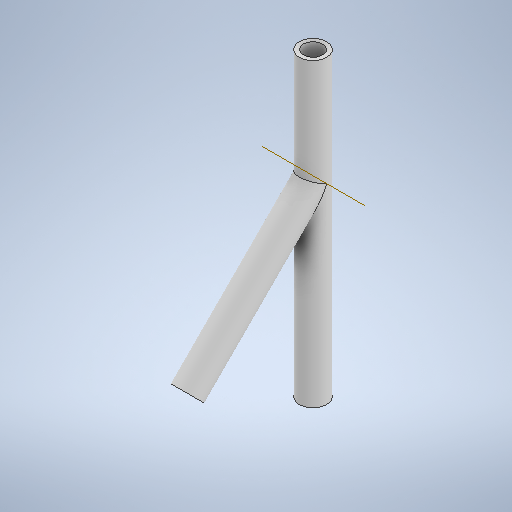
# Autodesk Inventor part: rurka
Saved by Autodesk Inventor 2025 (Build 290162000, 162)
## iProperties
Created: 2024-12-31
Part Number: rurka
Material: Ogólny
Document SubType Name: Modeling
Designer: Laptop
Density: 1 g/cm^3
Appearance: Domyślna
Author: Laptop
Autodesk Inventor part; units mm, degrees
ref_plane "YZ Plane" through (0, 0, 0) normal (1, 0, 0) x (0, 1, 0)
ref_plane "XZ Plane" through (0, 0, 0) normal (0, 1, 0) x (-1, 0, 0)
ref_plane "XY Plane" through (0, 0, 0) normal (0, 0, 1) x (1, 0, 0)
ref_plane "Płaszczyzna konstrukcyjna9" through (0, 0, 0) normal (0, -0.7071068, 0.7071068) x (1, 0, 0)
sketch "Szkic5" plane through (0, 0, 0) normal (0, -0.7071068, 0.7071068) x (1, 0, 0)
  circle A0 centre (0, 0) radius 5
  dimension "d1" = 10
  constraints: 1 centre point, 1 coincident
  measures "d1" diameter of A0
extrude "Wyciągnięcie proste1" add sketch "Szkic5" along normal blind 65
sketch "Szkic6" plane through (0, 0, 0) normal (0, 1, 0) x (-1, 0, 0)
  circle A0 centre (0, 0) radius 5
  dimension "d4" = 10
  constraints: 1 centre point, 1 coincident
  measures "d4" diameter of A0
extrude "Wyciągnięcie proste2" add sketch "Szkic6" along normal mid plane 140
sketch "Szkic8" plane through (0, -45.9619, 45.9619) normal (0, -0.7071068, 0.7071068) x (1, 0, 0)
  circle A0 centre (0, 0) radius 5 projected
  circle A1 centre (0, 0) radius 3.5
  dimension "d8" = 7
  constraints: 1 centre point, 1 coincident
  measures "d8" diameter of A1
extrude "Wyciągnięcie proste3" cut sketch "Szkic8" against normal blind 60 contours A1
sketch "Szkic9" plane through (0, 70, 0) normal (0, 1, 0) x (1, 0, 0)
  circle A0 centre (0, 0) radius 3.5
  dimension "d8" = 7
  dimension "d11" = 7
  constraints: 1 centre point, 1 coincident
  measures "d11" diameter of A0
extrude "Wyciągnięcie proste4" cut sketch "Szkic9" against normal blind 80
sketch "Szkic10" plane through (0, 70, 0) normal (0, 1, 0) x (1, 0, 0)
  arc A0 (-5, 0) -> (5, 0) centre (0, 0) ccw projected
  circle A1 centre (0, 0) radius 5
  point P0 (5, 0)
  dimension "d14" = 10
  constraints: 1 centre point, 1 coincident
  measures "d14" diameter of A1
extrude "Wyciągnięcie proste5" cut sketch "Szkic10" against normal blind 30
